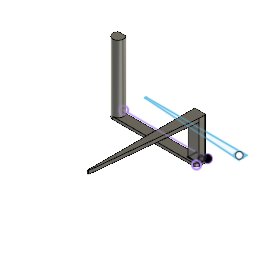
Chain aligner v6 (Autodesk Fusion 360 design; units mm, degrees)
Autodesk Fusion 360 part; units mm, degrees
sketch "Sketch1" plane through (0, 0, 0) normal (0, 0, 1) x (1, 0, 0)
  circle A0 centre (0, 0) radius 9.75
  line L0 (0, 9.75) -> (150, 9.75)
  line L1 (0, -9.75) -> (150, -9.75)
  line L2 (150, -9.75) -> (150, 9.75)
  dimension "d3" = 19.5
  dimension "d7" = 150
  dimension "d8" = 150
  constraint coincident A0.centre origin
  constraint coincident A0 L0.start
  constraint horizontal L0
  constraint tangent A0 L0
  constraint coincident A0 L1.start
  constraint horizontal L1
  constraint tangent A0 L1
  measures "d3" diameter of A0
  measures "d7" distance of L0.start L0.end
  measures "d8" distance of L1.start L1.end
extrude "Extrude1" add sketch "Sketch1" along normal blind 120 contours A0 makes body 1
extrude "Extrude2" add sketch "Sketch1" against normal blind 5 bodies 1
sketch "Sketch2" plane through (0, 0, 0) normal (0, 0, 1) x (1, 0, 0)
  line L0 (0, 9.75) -> (150, 9.75)
  line L1 (150, -9.75) -> (150, 9.75)
  circle A0 centre (145, 4.75) radius 5
  line L2 (0, 50) -> (180, 50)
  line L3 (180, 50) -> (180, 36)
  line L4 (0, 50) -> (0, 48)
  line L5 (0, 48) -> (180, 36)
  circle A1 centre (173.2331, 43.2331) radius 6.7669
  circle A2 centre (173.2331, 43.2331) radius 5.15
  line L6 (150, 9.75) -> (130, 9.75)
  line L7 (130, 9.75) -> (130, -5.25)
  line L8 (130, -5.25) -> (150, -5.25)
  line L9 (150, -5.25) -> (150, 9.75)
  dimension "d12" = 5
  dimension "d19" = 180
  dimension "d20" = 14
  dimension "d21" = 2
  dimension "d22" = 10.3
  dimension "d25" = 20
  dimension "d26" = 15
  constraint tangent L0 A0
  constraint tangent L1 A0
  constraint horizontal L2
  constraint perpendicular L2 L3
  constraint vertical L4
  constraint tangent L2 A1
  constraint tangent L3 A1
  constraint tangent L5 A1
  constraint concentric A1 A2
  constraint horizontal L6
  constraint vertical L7
  constraint horizontal L8
  constraint vertical L9
  constraint coincident L0.end L1.end
  measures "d12" radius of A0
  measures "d19" distance of L2.start L2.end
  measures "d20" distance of L2.end L3.end
  measures "d21" distance of L2.start L4.end
  measures "d22" diameter of A2
  measures "d25" distance of L0.end L6.end
  measures "d26" distance of L0.end L8.end
fillet "Fillet1" radius 5 2 edges at (150, 9.75, -2.5) (150, -9.75, -2.5) on bodies 1
extrude "Extrude8" add sketch "Sketch2" along normal blind 70 contours L0 L1 A0 L6 L7 L8 L9 | A0 bodies 1
sketch "Sketch5" plane through (0, -5.25, 0) normal (0, -1, 0) x (1, 0, 0)
  line L0 (130, 0) -> (149.9749, 0)
  line L1 (149.9749, 0) -> (150, 0)
  line L2 (150, 0) -> (150, 70)
  line L3 (150, 70) -> (130, 70)
  line L4 (130, 70) -> (130, 0)
  line L5 (150, 70) -> (130, 70)
  line L6 (130, 70) -> (130, 63.7)
  line L7 (130, 63.7) -> (150, 63.7)
  line L8 (150, 63.7) -> (150, 70)
  dimension "d37" = 6.3
  constraint horizontal L5
  constraint vertical L6
  constraint horizontal L7
  constraint vertical L8
  constraint coincident L4 L6.end
  constraint coincident L2.end L3.start
  measures "d37" distance of L2.end L7.end
extrude "Extrude9" add sketch "Sketch5" along normal blind 180 contours L2 L3 L4 L5 L6 L7 L8 bodies 1
chamfer "Chamfer2" distance 18 distance2 180 1 edges at (150, -185.25, 66.85) measured on face at (136.6667, -185.25, 67.9) on bodies 1
ref_plane "WorkPlane1" through (72.5, 7.25, 32.5) normal (0, 1, 0) x (1, 0, 0)
split "Split1" by plane through (72.5, 7.25, 32.5) normal (0, 1, 0) bodies 1 makes body 2 at (140, 9.75, 21.6667)
hidden bodies 2
equation "axleid = 19.50 mm"
equation "beamlength = 180 mm"
equation "d3 = axleid"
equation "linkinner = 6.3 mm"
equation "d7 = beamheight"
equation "d8 = beamheight"
equation "beamheight = 150 mm"
equation "d19 = beamlength"
equation "d20 = 10 mm + 2 mm + 2 mm"
equation "d37 = linkinner"
equation "d38 = beamlength"
equation "d41 = beamlength"
equation "d42 = -cutdepth"
equation "cutdepth = 2.5 mm"
named bodies: "pivot", "pivot (1)"
